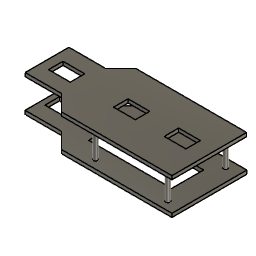
secondbody_prototype2 (Autodesk Fusion 360 design; units mm, degrees)
Autodesk Fusion 360 part; units mm, degrees
sketch "Sketch1" plane through (0, 0, 0) normal (0, 0, 1) x (1, 0, 0)
  line L0 (87.5, 51.8231) -> (-87.5, 51.8231)
  line L1 (-87.5, 51.8231) -> (-87.5, -51.8231)
  line L2 (-87.5, -51.8231) -> (87.5, -51.8231)
  line L3 (87.5, -51.8231) -> (87.5, 51.8231)
  line L4 (87.5, 51.8231) -> (-87.5, -51.8231) construction
  line L5 (-87.5, 51.8231) -> (87.5, -51.8231) construction
  line L6 (-87.5, 30.7122) -> (-137.5, 30.7122)
  line L7 (-137.5, 30.7122) -> (-137.5, -30)
  line L8 (-137.5, -30) -> (-87.5, -30)
  line L9 (-87.5, -30) -> (-87.5, 30.7122)
  dimension "d1" = 175
  dimension "d2" = 50
  constraint horizontal L0
  constraint perpendicular L0 L1
  constraint parallel L0 L2
  constraint parallel L1 L3
  constraint coincident L4 origin
  constraint coincident L5 origin
  constraint horizontal L6
  constraint vertical L7
  constraint horizontal L8
  constraint vertical L9
  constraint coincident L1 L6.start
  measures "d1" distance of L1.end L2.end
  measures "d2" distance of L6.start L6.end
extrude "Extrude1" add sketch "Sketch1" along normal blind 4 makes body 1
chamfer "Chamfer1" distance 21.8 angle 45 1 edges at (-87.5, -51.8231, 2) on bodies 1
chamfer "Chamfer2" distance 21.11 angle 45 1 edges at (-87.5, 51.8231, 2) on bodies 1
sketch "Sketch2" plane through (0, 0, 4) normal (0, 0, 1) x (-1, 0, 0)
  line L0 (66.39, -51.8231) -> (87.5, -30.7131)
  line L1 (87.5, -30.7131) -> (87.5, -30.7122)
  line L2 (87.5, -30.7122) -> (137.5, -30.7122)
  line L3 (137.5, -30.7122) -> (137.5, 30)
  line L4 (137.5, 30) -> (87.5, 30)
  line L5 (87.5, 30) -> (87.5, 30.0231)
  line L6 (87.5, 30.0231) -> (65.7, 51.8231)
  line L7 (65.7, 51.8231) -> (-87.5, 51.8231)
  line L8 (-87.5, 51.8231) -> (-87.5, -51.8231)
  line L9 (-87.5, -51.8231) -> (66.39, -51.8231)
  line L10 (130, 10) -> (90, 10)
  line L11 (90, 10) -> (90, -10)
  line L12 (90, -10) -> (130, -10)
  line L13 (130, -10) -> (130, 10)
  line L14 (130, 10) -> (90, -10) construction
  line L15 (90, 10) -> (130, -10) construction
  point P0 (110, 0)
  dimension "d7" = 40
  dimension "d8" = 20
  constraint horizontal L10
  constraint perpendicular L10 L11
  constraint parallel L10 L12
  constraint parallel L11 L13
  constraint coincident L14 P0
  constraint coincident L15 P0
  measures "d7" distance of L11.end L12.end
  measures "d8" distance of L10.end L11.end
extrude "Extrude2" cut sketch "Sketch2" against normal blind 70 contours L10 L11 L12 L13 bodies 1
sketch "Sketch3" plane through (0, 0, 4) normal (0, 0, 1) x (-1, 0, 0)
  line L0 (90, 10) -> (130, 10)
  line L1 (130, 10) -> (130, -10)
  line L2 (130, -10) -> (90, -10)
  line L3 (90, -10) -> (90, 10)
  line L4 (66.39, -51.8231) -> (87.5, -30.7131)
  line L5 (87.5, -30.7131) -> (87.5, -30.7122)
  line L6 (87.5, -30.7122) -> (137.5, -30.7122)
  line L7 (137.5, -30.7122) -> (137.5, 30)
  line L8 (137.5, 30) -> (87.5, 30)
  line L9 (87.5, 30) -> (87.5, 30.0231)
  line L10 (87.5, 30.0231) -> (65.7, 51.8231)
  line L11 (65.7, 51.8231) -> (-87.5, 51.8231)
  line L12 (-87.5, 51.8231) -> (-87.5, -51.8231)
  line L13 (-87.5, -51.8231) -> (66.39, -51.8231)
  line L14 (-57.5, -22) -> (57.5, -22)
  line L15 (57.5, -22) -> (57.5, 22)
  line L16 (57.5, 22) -> (-57.5, 22)
  line L17 (-57.5, 22) -> (-57.5, -22)
  line L18 (-57.5, -22) -> (57.5, 22) construction
  line L19 (57.5, -22) -> (-57.5, 22) construction
  dimension "d11" = 115
  dimension "d12" = 44
  constraint horizontal L14
  constraint perpendicular L14 L15
  constraint parallel L14 L16
  constraint parallel L15 L17
  constraint coincident L18 origin
  constraint coincident L19 origin
  measures "d11" distance of L15.end L16.end
  measures "d12" distance of L14.end L15.end
extrude "Extrude3" cut sketch "Sketch3" against normal blind 50 contours L14 L15 L16 L17 bodies 1
sketch "Sketch4" plane through (0, 0, 4) normal (0, 0, 1) x (-1, 0, 0)
  line L0 (57.5, -22) -> (-57.5, -22)
  line L1 (-57.5, -22) -> (-57.5, 22)
  line L2 (-57.5, 22) -> (57.5, 22)
  line L3 (57.5, 22) -> (57.5, -22)
  line L4 (90, 10) -> (130, 10)
  line L5 (130, 10) -> (130, -10)
  line L6 (130, -10) -> (90, -10)
  line L7 (90, -10) -> (90, 10)
  line L8 (66.39, -51.8231) -> (87.5, -30.7131)
  line L9 (87.5, -30.7131) -> (87.5, -30.7122)
  line L10 (87.5, -30.7122) -> (137.5, -30.7122)
  line L11 (137.5, -30.7122) -> (137.5, 30)
  line L12 (137.5, 30) -> (87.5, 30)
  line L13 (87.5, 30) -> (87.5, 30.0231)
  line L14 (87.5, 30.0231) -> (65.7, 51.8231)
  line L15 (65.7, 51.8231) -> (-87.5, 51.8231)
  line L16 (-87.5, 51.8231) -> (-87.5, -51.8231)
  line L17 (-87.5, -51.8231) -> (66.39, -51.8231)
  circle A0 centre (30, -40) radius 3
  circle A1 centre (30, 40) radius 3
  circle A2 centre (-70, 40) radius 3
  circle A3 centre (-70, -40) radius 3
  dimension "d15" = 6
  dimension "d16" = 6
  dimension "d17" = 6
  dimension "d18" = 6
  measures "d15" diameter of A0
  measures "d16" diameter of A1
  measures "d17" diameter of A2
  measures "d18" diameter of A3
extrude "Extrude4" add sketch "Sketch4" along normal blind 40 contours A0 | A1 | A2 | A3 bodies 1
sketch "Sketch5" plane through (0, 0, 44) normal (0, 0, 1) x (-1, 0, 0)
  circle A0 centre (30, 40) radius 3
  line L0 (-87.357, -51.7293) -> (87.357, -51.7293)
  line L1 (87.357, -51.7293) -> (87.357, 51.7293)
  line L2 (87.357, 51.7293) -> (-87.357, 51.7293)
  line L3 (-87.357, 51.7293) -> (-87.357, -51.7293)
  line L4 (-87.357, -51.7293) -> (87.357, 51.7293) construction
  line L5 (87.357, -51.7293) -> (-87.357, 51.7293) construction
  line L6 (87.357, -30.8475) -> (137.7031, -30.8475)
  line L7 (137.7031, -30.8475) -> (137.7031, 29.6713)
  line L8 (137.7031, 29.6713) -> (87.357, 29.6713)
  line L9 (87.357, 29.6713) -> (87.357, -30.8475)
  constraint horizontal L0
  constraint perpendicular L0 L1
  constraint parallel L0 L2
  constraint parallel L1 L3
  constraint coincident L4 origin
  constraint coincident L5 origin
  constraint horizontal L6
  constraint vertical L7
  constraint horizontal L8
  constraint vertical L9
  constraint coincident L1 L6.start
extrude "Extrude5" add sketch "Sketch5" along normal blind 5 separate body makes body 2
sketch "Sketch6" plane through (0, 0, 44) normal (0, 0, 1) x (-1, 0, 0)
  circle A0 centre (30, 40) radius 3
  circle A1 centre (30, 40) radius 3
  dimension "d23" = 6
  constraint concentric A0 A1
  measures "d23" diameter of A1
extrude "Extrude6" add sketch "Sketch6" along normal blind 5 bodies 1 2
chamfer "Chamfer3" distance 22.05 angle 45 1 edges at (-87.357, -51.7293, 46.5) on bodies 1
chamfer "Chamfer4" distance 20.88 angle 45 1 edges at (-87.357, 51.7293, 46.5) on bodies 1
sketch "Sketch7" plane through (0, 0, 49) normal (0, 0, 1) x (-1, 0, 0)
  line L0 (66.477, -51.7293) -> (87.357, -30.8493)
  line L1 (87.357, -30.8493) -> (87.357, -30.8475)
  line L2 (87.357, -30.8475) -> (137.7031, -30.8475)
  line L3 (137.7031, -30.8475) -> (137.7031, 29.6713)
  line L4 (137.7031, 29.6713) -> (87.357, 29.6713)
  line L5 (87.357, 29.6713) -> (87.357, 29.6793)
  line L6 (87.357, 29.6793) -> (65.307, 51.7293)
  line L7 (65.307, 51.7293) -> (-87.357, 51.7293)
  line L8 (-87.357, 51.7293) -> (-87.357, -51.7293)
  line L9 (-87.357, -51.7293) -> (66.477, -51.7293)
  line L10 (-35, 10) -> (-65, 10)
  line L11 (-65, 10) -> (-65, -10)
  line L12 (-65, -10) -> (-35, -10)
  line L13 (-35, -10) -> (-35, 10)
  line L14 (-35, 10) -> (-65, -10) construction
  line L15 (-65, 10) -> (-35, -10) construction
  line L16 (35, 10) -> (5, 10)
  line L17 (5, 10) -> (5, -10)
  line L18 (5, -10) -> (35, -10)
  line L19 (35, -10) -> (35, 10)
  line L20 (35, 10) -> (5, -10) construction
  line L21 (5, 10) -> (35, -10) construction
  line L22 (125, 10) -> (95, 10)
  line L23 (95, 10) -> (95, -10)
  line L24 (95, -10) -> (125, -10)
  line L25 (125, -10) -> (125, 10)
  line L26 (125, 10) -> (95, -10) construction
  line L27 (95, 10) -> (125, -10) construction
  point P0 (-50, 0)
  point P1 (20, 0)
  point P2 (110, 0)
  dimension "d28" = 30
  dimension "d29" = 20
  dimension "d30" = 30
  dimension "d31" = 20
  dimension "d32" = 30
  dimension "d33" = 20
  constraint horizontal L10
  constraint perpendicular L10 L11
  constraint parallel L10 L12
  constraint parallel L11 L13
  constraint coincident L14 P0
  constraint coincident L15 P0
  constraint horizontal L16
  constraint perpendicular L16 L17
  constraint parallel L16 L18
  constraint parallel L17 L19
  constraint coincident L20 P1
  constraint coincident L21 P1
  constraint horizontal L22
  constraint perpendicular L22 L23
  constraint parallel L22 L24
  constraint parallel L23 L25
  constraint coincident L26 P2
  constraint coincident L27 P2
  measures "d28" distance of L11.end L12.end
  measures "d29" distance of L10.end L11.end
  measures "d30" distance of L17.end L18.end
  measures "d31" distance of L16.end L17.end
  measures "d32" distance of L23.end L24.end
  measures "d33" distance of L22.end L23.end
extrude "Extrude7" cut sketch "Sketch7" against normal blind 15 contours L10 L11 L12 L13 | L16 L17 L18 L19 | L22 L23 L24 L25 bodies 1
move_face "OffsetFaces1" offset 1 1 faces at (26.2033, 41.882, 0) on bodies 1
